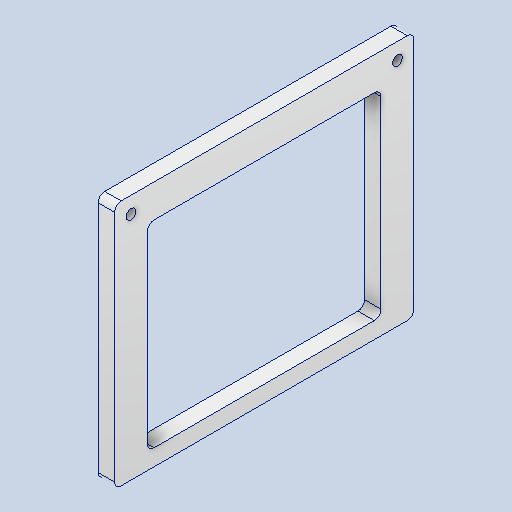
# Autodesk Inventor part: base_weel-v2-Plate-6
Saved by Autodesk Inventor 2025.2 (Build 292293000, 293)
## iProperties
Created: 2025-01-14
Part Number: base_weel-v2-Plate-6
Material: アルミニウム 6061
Document SubType Name: Modeling
Designer: haruy
Density: 2.7 g/cm^3
Appearance: アルミニウム - フラット
Author: haruy
Autodesk Inventor part; units mm, degrees
ref_plane "YZ Plane" through (0, 0, 0) normal (1, 0, 0) x (0, 1, 0)
ref_plane "XZ Plane" through (0, 0, 0) normal (0, 1, 0) x (-1, 0, 0)
ref_plane "XY Plane" through (0, 0, 0) normal (0, 0, 1) x (1, 0, 0)
sketch "スケッチ1" plane through (0, 0, 0) normal (1, 0, 0) x (0, 1, 0)
  line L0 (-222.6453, 335.6671) -> (407.3547, 335.6671)
  line L1 (407.3547, 335.6671) -> (407.3547, -294.3329)
  line L2 (407.3547, -294.3329) -> (-222.6453, -294.3329)
  line L3 (-222.6453, -294.3329) -> (-222.6453, 335.6671)
  line L4 (-222.6453, 335.6671) -> (407.3547, -294.3329) construction
  line L5 (407.3547, 335.6671) -> (-222.6453, -294.3329) construction
  line L6 (-202.6453, 238.6671) -> (-202.6453, -181.3329)
  line L7 (-202.6453, -181.3329) -> (-222.6453, -181.3329)
  line L8 (-222.6453, -181.3329) -> (-222.6453, 230.6671)
  line L9 (334.3547, 335.6671) -> (-149.6453, 335.6671)
  line L10 (-149.6453, 335.6671) -> (-149.6453, 315.6671)
  line L11 (-149.6453, 315.6671) -> (334.3547, 315.6671)
  line L12 (334.3547, 315.6671) -> (334.3547, 335.6671)
  line L13 (-202.6453, 238.6671) -> (-202.6453, 335.6671)
  line L14 (92.3547, 20.6671) -> (-864.2426, 20.6671)
  circle A0 centre (92.3547, 20.6671) radius 400
  line L15 (-237.6453, 45.6671) -> (-287.6453, 45.6671)
  line L16 (-287.6453, 45.6671) -> (-287.6453, -4.3329)
  line L17 (-287.6453, -4.3329) -> (-237.6453, -4.3329)
  line L18 (-237.6453, -4.3329) -> (-237.6453, 45.6671)
  line L19 (92.3547, 20.6671) -> (92.3547, -610.2507)
  line L20 (-222.6453, 60.6671) -> (-302.6453, 60.6671) construction
  line L21 (-302.6453, 60.6671) -> (-302.6453, 50.6671)
  line L22 (-302.6453, 50.6671) -> (-222.6453, 50.6671)
  line L23 (-222.6453, 50.6671) -> (-222.6453, 60.6671)
  line L24 (-302.6453, 50.6671) -> (-292.6453, 50.6671)
  line L25 (-292.6453, 50.6671) -> (-292.6453, 20.6671)
  line L26 (-292.6453, 20.6671) -> (-302.6453, 20.6671)
  line L27 (-302.6453, 20.6671) -> (-302.6453, 50.6671)
  line L28 (387.3547, 222.6671) -> (407.3547, 222.6671)
  line L29 (407.3547, 222.6671) -> (407.3547, -181.3329)
  line L30 (407.3547, -181.3329) -> (387.3547, -181.3329)
  line L31 (387.3547, -181.3329) -> (387.3547, 222.6671)
  line L32 (-129.8635, -294.3329) -> (334.3547, -294.3329)
  line L33 (334.3547, -294.3329) -> (334.3547, -274.3329)
  line L34 (334.3547, -274.3329) -> (-149.6453, -274.3329)
  line L35 (407.3547, 335.6671) -> (92.3547, 20.6671)
  line L36 (407.3547, 145.6671) -> (407.3547, 165.6671)
  circle A1 centre (604.3547, 20.6671) radius 122.5
  circle A2 centre (272.0452, 20.6671) radius 600
  circle A3 centre (634.0363, 20.6671) radius 200
  circle A4 centre (92.3547, 20.6671) radius 10
  arc A5 (92.3547, 170.6671) -> (92.3547, -129.3329) centre (92.3547, 20.6671) ccw
  arc A6 (92.3547, 160.6671) -> (92.3547, -119.3329) centre (92.3547, 20.6671) ccw
  line L37 (-53.9724, 53.6575) -> (-44.2173, 51.4581)
  line L38 (-45.2265, 58.3488) -> (-48.0856, 45.6671)
  line L39 (-48.0856, 45.6671) -> (-52.9632, 46.7668)
  line L40 (-52.9632, 46.7668) -> (-50.104, 59.4485)
  line L41 (-50.104, 59.4485) -> (-45.2265, 58.3488)
  arc A7 (63.2246, 162.7109) -> (63.2246, -121.3767) centre (92.3547, 20.6671) ccw
  circle A8 centre (-59.1356, 59.9471) radius 6.5
  circle A9 centre (-36.6854, 54.8855) radius 6.5 construction
  circle A10 centre (-36.6854, 54.8855) radius 1.5 construction
  circle A11 centre (-59.1356, 59.9471) radius 1.5
  line L42 (62.1879, 43.1671) -> (-81.7815, 43.1671)
  line L43 (-81.7815, 43.1671) -> (-81.7815, 28.1671)
  line L44 (-81.7815, 28.1671) -> (62.1879, 28.1671)
  line L45 (62.1879, 28.1671) -> (62.1879, 43.1671)
  line L46 (-53.9724, -12.3232) -> (-44.2173, -10.1239)
  line L47 (-45.2265, -17.0146) -> (-48.0856, -4.3329)
  line L48 (-48.0856, -4.3329) -> (-52.9632, -5.4326)
  line L49 (-52.9632, -5.4326) -> (-50.104, -18.1142)
  line L50 (-50.104, -18.1142) -> (-45.2265, -17.0146)
  circle A12 centre (-59.1356, -18.6128) radius 6.5
  circle A13 centre (-36.6854, -13.5513) radius 6.5 construction
  circle A14 centre (-36.6854, -13.5513) radius 1.5 construction
  circle A15 centre (-59.1356, -18.6128) radius 1.5
  line L51 (62.1879, -1.8329) -> (-81.7815, -1.8329)
  line L52 (-81.7815, -1.8329) -> (-81.7815, 13.1671)
  line L53 (-81.7815, 13.1671) -> (62.1879, 13.1671)
  line L54 (62.1879, 13.1671) -> (62.1879, -1.8329)
  line L55 (-59.1356, 59.9471) -> (-36.6854, 54.8855) construction
  line L56 (-36.6854, 54.8855) -> (-37.2352, 52.4467) construction
  line L57 (-37.2352, 52.4467) -> (-59.6855, 57.5083) construction
  line L58 (-59.6855, 57.5083) -> (-59.1356, 59.9471) construction
  line L59 (-36.6854, 54.8855) -> (-59.1356, 59.9471) construction
  line L60 (-59.1356, 59.9471) -> (-58.5858, 62.3858) construction
  line L61 (-58.5858, 62.3858) -> (-36.1355, 57.3243) construction
  line L62 (-36.1355, 57.3243) -> (-36.6854, 54.8855) construction
  line L63 (-36.1355, 57.3243) -> (-37.2352, 52.4467) construction
  line L64 (-37.2352, 52.4467) -> (-25.529, 49.8075) construction
  line L65 (-25.529, 49.8075) -> (-24.4294, 54.6851) construction
  line L66 (-24.4294, 54.6851) -> (-36.1355, 57.3243) construction
  line L67 (-58.5858, 62.3858) -> (-59.6855, 57.5083) construction
  line L68 (-59.6855, 57.5083) -> (-71.3917, 60.1475) construction
  line L69 (-71.3917, 60.1475) -> (-70.292, 65.0251) construction
  line L70 (-70.292, 65.0251) -> (-58.5858, 62.3858) construction
  line L71 (-62.9135, 65.9243) -> (-36.5865, 59.9887)
  line L72 (-36.5865, 59.9887) -> (-39.8855, 45.356)
  line L73 (-39.8855, 45.356) -> (-66.2126, 51.2916)
  line L74 (-66.2126, 51.2916) -> (-62.9135, 65.9243)
  line L75 (-62.9135, -24.5901) -> (-36.5865, -18.6545)
  line L76 (-36.5865, -18.6545) -> (-39.8855, -4.0218)
  line L77 (-39.8855, -4.0218) -> (-66.2126, -9.9574)
  line L78 (-66.2126, -9.9574) -> (-62.9135, -24.5901)
  arc A16 (-39.8855, 45.356) -> (-39.8855, -4.0218) centre (92.3547, 20.6671) ccw
  arc A17 (-66.2126, 51.2916) -> (-66.2126, -9.9574) centre (92.3547, 20.6671) ccw
  circle A18 centre (-60.1453, 35.6671) radius 1.25
  line L79 (-52.6453, 20.6671) -> (-52.6453, 95.4053)
  circle A19 centre (-45.1453, 35.6671) radius 1.25
  circle A20 centre (-60.1453, 5.6671) radius 1.25
  circle A21 centre (-45.1453, 5.6671) radius 1.25
  line L80 (92.3547, 20.6671) -> (92.3547, 160.6671)
  line L81 (92.3547, 20.6671) -> (44.4719, 152.2241)
  line L82 (92.3547, 160.6671) -> (92.3547, 170.6671)
  line L83 (-45.2298, 46.5609) -> (-41.9308, 61.1936)
  line L84 (-45.2298, -5.2267) -> (-41.9308, -19.8594)
  circle A22 centre (92.3547, 20.6671) radius 20
  line L85 (387.3547, 65.6671) -> (-202.6453, 65.6671)
  line L86 (-202.6453, 65.6671) -> (-202.6453, 45.6671)
  line L87 (-202.6453, 45.6671) -> (387.3547, 45.6671)
  line L88 (387.3547, 45.6671) -> (387.3547, 65.6671)
  line L89 (52.3547, 315.6671) -> (42.3547, 315.6671)
  line L90 (42.3547, 315.6671) -> (42.3547, 65.6671)
  line L91 (42.3547, 65.6671) -> (52.3547, 65.6671)
  line L92 (52.3547, 65.6671) -> (52.3547, 315.6671)
  line L93 (387.3547, -24.3329) -> (-202.6453, -24.3329)
  line L94 (-202.6453, -4.3329) -> (387.3547, -4.3329)
  line L95 (42.3547, -274.3329) -> (42.3547, -24.3329)
  line L96 (52.3547, -24.3329) -> (52.3547, -274.3329)
  line L97 (52.3547, 65.6671) -> (52.3547, -24.3329)
  line L98 (132.3547, 65.6671) -> (132.3547, -24.3329)
  circle A23 centre (112.3547, 55.6671) radius 1.5
  circle A24 centre (72.3547, 55.6671) radius 1.5
  circle A25 centre (112.3547, -14.3329) radius 1.5
  circle A26 centre (72.3547, -14.3329) radius 1.5
  circle A27 centre (47.3547, 145.6671) radius 1.5
  circle A28 centre (47.3547, 145.6671) radius 5
  circle A29 centre (-37.6453, 55.6671) radius 5
  circle A30 centre (-37.6453, 55.6671) radius 1.5
  line L99 (52.3547, 154.8312) -> (52.3547, 145.6671)
  line L100 (42.3547, 145.6671) -> (42.3547, 151.4341)
  line L101 (-45.395, 45.6671) -> (-35.2253, 51.2917)
  line L102 (-40.216, 65.6671) -> (-34.0112, 59.1013)
  circle A31 centre (47.3547, -104.3329) radius 1.5
  circle A32 centre (47.3547, -104.3329) radius 5
  circle A33 centre (-37.6453, -14.3329) radius 5
  circle A34 centre (-37.6453, -14.3329) radius 1.5
  line L103 (52.3547, -113.497) -> (52.3547, -104.3329)
  line L104 (42.3547, -104.3329) -> (42.3547, -110.0999)
  line L105 (-45.395, -4.3329) -> (-35.2253, -9.9575)
  line L106 (-40.216, -24.3329) -> (-34.0112, -17.7671)
  line L107 (-149.6453, -274.3329) -> (-149.6453, -294.3329)
  line L108 (334.3547, 335.6671) -> (314.3547, 335.6671)
  line L109 (314.3547, 335.6671) -> (314.3547, 315.6671)
  line L110 (314.3547, 315.6671) -> (334.3547, 315.6671)
  line L111 (334.3547, 315.6671) -> (334.3547, 335.6671)
  line L112 (334.3547, -294.3329) -> (314.3547, -294.3329)
  line L113 (314.3547, -294.3329) -> (314.3547, -274.3329)
  line L114 (314.3547, -274.3329) -> (334.3547, -274.3329)
  line L115 (334.3547, -274.3329) -> (334.3547, -294.3329)
  line L116 (289.3547, 315.6671) -> (387.3547, 217.6671)
  line L117 (387.3547, 217.6671) -> (376.7481, 207.0605)
  line L118 (376.7481, 207.0605) -> (278.7481, 305.0605)
  line L119 (278.7481, 305.0605) -> (289.3547, 315.6671)
  line L120 (289.3547, 315.6671) -> (289.3547, 335.6671)
  line L121 (290.2715, 314.7504) -> (279.6649, 304.1438)
  line L122 (290.625, 293.1836) -> (364.8712, 218.9374)
  line L123 (364.8712, 218.9374) -> (323.8591, 177.9252)
  line L124 (323.8591, 177.9252) -> (249.6128, 252.1714)
  line L125 (249.6128, 252.1714) -> (290.625, 293.1836)
  line L126 (383.256, 221.7658) -> (372.6494, 211.1592)
  line L127 (186.1172, 315.6671) -> (387.3547, 114.4295)
  line L128 (387.3547, 114.4295) -> (376.7481, 103.8229)
  line L129 (376.7481, 103.8229) -> (175.5105, 305.0605)
  line L130 (306.5349, 298.4869) -> (295.9283, 287.8803)
  line L131 (370.1745, 234.8473) -> (359.5679, 224.2407)
  circle A35 centre (292.0392, 302.376) radius 1.5
  circle A36 centre (306.1814, 288.2339) radius 1.5
  line L132 (278.7481, 305.0605) -> (268.1415, 315.6671)
  circle A37 centre (279.3547, 325.6671) radius 1.5
  circle A38 centre (269.3547, 325.6671) radius 1.5
  line L133 (264.3547, 335.6671) -> (264.3547, 315.6671)
  line L134 (186.1172, 315.6671) -> (186.1172, 315.6671)
  line L135 (186.1172, 315.6671) -> (186.1172, 335.6671)
  line L136 (175.5105, 305.0605) -> (164.9039, 315.6671)
  line L137 (161.1172, 335.6671) -> (161.1172, 315.6671)
  line L138 (376.7481, 207.0605) -> (387.3547, 196.4539)
  line L139 (387.3547, 217.6671) -> (407.3547, 217.6671)
  line L140 (387.3547, 114.4295) -> (387.3547, 114.4295)
  line L141 (376.7481, 103.8229) -> (387.3547, 93.2163)
  line L142 (-104.6453, 315.6671) -> (-202.6453, 217.6671)
  line L143 (-192.0387, 207.0605) -> (-94.0387, 305.0605)
  line L144 (-104.6453, 315.6671) -> (-104.6453, 335.6671)
  line L145 (-105.562, 314.7504) -> (-94.9554, 304.1438)
  line L146 (-180.1618, 218.9374) -> (-139.1496, 177.9252)
  line L147 (-64.9034, 252.1714) -> (-105.9156, 293.1836)
  line L148 (-198.5465, 221.7658) -> (-187.9399, 211.1592)
  line L149 (-1.4077, 315.6671) -> (-202.6453, 114.4295)
  line L150 (-202.6453, 114.4295) -> (-192.0387, 103.8229)
  line L151 (-192.0387, 103.8229) -> (9.1989, 305.0605)
  line L152 (9.1989, 305.0605) -> (-1.4077, 315.6671)
  line L153 (-121.8255, 298.4869) -> (-111.2189, 287.8803)
  line L154 (-94.0387, 305.0605) -> (-83.4321, 315.6671)
  line L155 (-79.6453, 335.6671) -> (-79.6453, 315.6671)
  line L156 (-1.4077, 315.6671) -> (-1.4077, 335.6671)
  line L157 (9.1989, 305.0605) -> (19.8055, 315.6671)
  line L158 (23.5923, 335.6671) -> (23.5923, 315.6671)
  line L159 (-192.0387, 207.0605) -> (-202.6453, 196.4539)
  line L160 (-202.6453, 217.6671) -> (-222.6453, 217.6671)
  line L161 (-192.0387, 103.8229) -> (-202.6453, 93.2163)
  line L162 (289.3547, -274.3329) -> (387.3547, -176.3329)
  line L163 (376.7481, -165.7263) -> (278.7481, -263.7263)
  line L164 (290.2715, -273.4161) -> (279.6649, -262.8095)
  line L165 (383.256, -180.4316) -> (372.6494, -169.825)
  line L166 (186.1172, -274.3329) -> (387.3547, -73.0953)
  line L167 (387.3547, -73.0953) -> (376.7481, -62.4887)
  line L168 (376.7481, -62.4887) -> (175.5105, -263.7263)
  line L169 (175.5105, -263.7263) -> (186.1172, -274.3329)
  line L170 (-1.4077, -274.3329) -> (-202.6453, -73.0953)
  line L171 (9.1989, -263.7263) -> (-1.4077, -274.3329)
  line L172 (-192.0387, -62.4887) -> (9.1989, -263.7263)
  line L173 (-202.6453, -73.0953) -> (-192.0387, -62.4887)
  line L174 (-192.0387, -165.7263) -> (-94.0387, -263.7263)
  line L175 (-104.6453, -274.3329) -> (-202.6453, -176.3329)
  line L176 (-105.562, -273.4161) -> (-94.9554, -262.8095)
  line L177 (-121.8255, -257.1527) -> (-111.2189, -246.5461)
  line L178 (-198.5465, -180.4316) -> (-187.9399, -169.825)
  line L179 (334.3547, 315.6671) -> (314.3547, 315.6671)
  arc A39 (92.3547, 106.6671) -> (92.3547, -65.3329) centre (92.3547, 20.6671) ccw construction
  circle A40 centre (1.4881, 69.1671) radius 21
  circle A41 centre (92.3547, 20.6671) radius 124
  circle A42 centre (1.4881, 69.1671) radius 17
  arc A43 (132.8499, 96.5364) -> (92.3547, 106.6671) centre (92.3547, 20.6671) ccw construction
  line L180 (52.3547, 65.6671) -> (42.3547, 65.6671)
  line L181 (42.3547, 65.6671) -> (42.3547, -24.3329)
  line L182 (42.3547, -24.3329) -> (52.3547, -24.3329)
  line L183 (52.3547, -24.3329) -> (52.3547, 65.6671)
  line L184 (52.3547, 315.6671) -> (42.3547, 315.6671)
  line L185 (42.3547, 315.6671) -> (42.3547, 335.6671)
  line L186 (42.3547, 335.6671) -> (52.3547, 335.6671)
  line L187 (52.3547, 335.6671) -> (52.3547, 315.6671)
  line L188 (52.3547, -274.3329) -> (42.3547, -274.3329)
  line L189 (42.3547, -274.3329) -> (42.3547, -294.3329)
  line L190 (42.3547, -294.3329) -> (52.3547, -294.3329)
  line L191 (52.3547, -294.3329) -> (52.3547, -274.3329)
  line L192 (142.3547, 315.6671) -> (142.3547, 65.6671)
  line L193 (132.3547, 65.6671) -> (132.3547, 315.6671)
  line L194 (142.3547, -274.3329) -> (142.3547, -24.3329)
  line L195 (132.3547, -24.3329) -> (132.3547, -274.3329)
  line L196 (142.3547, 65.6671) -> (142.3547, -24.3329)
  line L197 (132.3547, -24.3329) -> (132.3547, 65.6671)
  line L198 (142.3547, 315.6671) -> (142.3547, 335.6671)
  line L199 (132.3547, 335.6671) -> (132.3547, 315.6671)
  line L200 (142.3547, -274.3329) -> (142.3547, -294.3329)
  line L201 (132.3547, -294.3329) -> (132.3547, -274.3329)
  line L202 (51.9456, 143.6861) -> (57.3547, 156.2215)
  line L203 (43.613, 142.3505) -> (37.3547, 149.411)
  line L204 (51.9456, -102.3519) -> (57.3547, -114.8873)
  line L205 (43.613, -101.0163) -> (37.3547, -108.0768)
  arc A44 (132.8499, 96.5364) -> (51.8596, -55.2021) centre (92.3547, 20.6671) ccw
  circle A45 centre (92.3547, 20.6671) radius 86 construction
  circle A46 centre (92.3547, 20.6671) radius 78.5
  circle A47 centre (47.3547, 78.6671) radius 1.5
  circle A48 centre (47.3547, 78.6671) radius 5
  circle A49 centre (137.3547, 78.6671) radius 5
  circle A50 centre (137.3547, 78.6671) radius 1.5
  line L206 (138.9096, 73.915) -> (147.3547, 76.6783)
  line L207 (132.6797, 76.8939) -> (127.3547, 90.9327)
  line L208 (142.3547, 81.1836) -> (142.3547, 90.6385)
  arc A51 (142.3547, 90.6385) -> (132.8499, 96.5364) centre (92.3547, 20.6671) ccw
  line L209 (52.0297, 76.8939) -> (57.3547, 90.9327)
  line L210 (45.7999, 73.915) -> (37.3547, 76.6783)
  circle A52 centre (47.3547, -37.3329) radius 1.5
  circle A53 centre (47.3547, -37.3329) radius 5
  line L211 (52.0297, -35.5596) -> (57.3547, -49.5985) construction
  line L212 (45.7999, -32.5808) -> (37.3547, -35.344)
  line L213 (52.3547, -46.8773) -> (52.3547, -55.4643)
  arc A54 (51.8288, -55.1857) -> (52.3547, -55.4643) centre (92.3547, 20.6671) ccw
  line L214 (52.3547, -55.4643) -> (52.3547, -37.3329)
  line L215 (315.0202, 290.0016) -> (304.4136, 279.395)
  line L216 (387.3547, 217.6671) -> (407.3547, 217.6671)
  line L217 (386.438, 218.5839) -> (375.8314, 207.9773)
  circle A55 centre (374.0636, 220.3516) radius 1.5
  circle A56 centre (359.9215, 234.4938) radius 1.5
  circle A57 centre (397.3547, 207.6671) radius 1.5
  circle A58 centre (397.3547, 197.6671) radius 1.5
  line L218 (407.3547, 192.6671) -> (387.3547, 192.6671)
  line L219 (361.6893, 243.3326) -> (351.0827, 232.726)
  circle A59 centre (176.1172, 325.6671) radius 1.5
  circle A60 centre (166.1172, 325.6671) radius 1.5
  line L220 (290.2715, 314.7504) -> (187.0339, 314.7504)
  line L221 (279.6649, 304.1438) -> (176.4273, 304.1438)
  line L222 (187.0339, 314.7504) -> (176.4273, 304.1438)
  circle A61 centre (188.8017, 302.376) radius 1.5
  circle A62 centre (202.9438, 288.2339) radius 1.5
  line L223 (211.7826, 290.0016) -> (201.176, 279.395)
  line L224 (387.3547, 114.4295) -> (407.3547, 114.4295)
  line L225 (407.3547, 89.4295) -> (387.3547, 89.4295)
  circle A63 centre (397.3547, 104.4295) radius 1.5
  circle A64 centre (397.3547, 94.4295) radius 1.5
  line L226 (386.438, 115.3463) -> (375.8314, 104.7397)
  circle A65 centre (374.0636, 117.114) radius 1.5
  circle A66 centre (359.9215, 131.2562) radius 1.5
  line L227 (361.6893, 140.095) -> (351.0827, 129.4884)
  line L228 (-104.6453, 315.6671) -> (-104.6453, 335.6671)
  line L229 (-105.562, 314.7504) -> (-94.9554, 304.1438)
  line L230 (-121.8255, 298.4869) -> (-111.2189, 287.8803)
  circle A67 centre (-107.3298, 302.376) radius 1.5
  circle A68 centre (-121.4719, 288.2339) radius 1.5
  circle A69 centre (-94.6453, 325.6671) radius 1.5
  circle A70 centre (-84.6453, 325.6671) radius 1.5
  line L231 (-79.6453, 335.6671) -> (-79.6453, 315.6671)
  line L232 (-1.4077, 315.6671) -> (-1.4077, 335.6671)
  line L233 (23.5923, 335.6671) -> (23.5923, 315.6671)
  line L234 (-202.6453, 217.6671) -> (-222.6453, 217.6671)
  line L235 (-130.3107, 290.0016) -> (-119.7041, 279.395)
  line L236 (-176.9798, 243.3326) -> (-166.3732, 232.726)
  circle A71 centre (-175.212, 234.4938) radius 1.5
  circle A72 centre (-189.3542, 220.3516) radius 1.5
  line L237 (-201.7285, 218.5839) -> (-191.1219, 207.9773)
  line L238 (-222.6453, 192.6671) -> (-202.6453, 192.6671)
  circle A73 centre (-212.6453, 197.6671) radius 1.5
  circle A74 centre (-212.6453, 207.6671) radius 1.5
  circle A75 centre (8.5923, 325.6671) radius 1.5
  circle A76 centre (18.5923, 325.6671) radius 1.5
  line L239 (-2.3244, 314.7504) -> (8.2822, 304.1438)
  circle A77 centre (-4.0922, 302.376) radius 1.5
  circle A78 centre (-18.2343, 288.2339) radius 1.5
  line L240 (-27.0731, 290.0016) -> (-16.4665, 279.395)
  line L241 (-202.6453, 114.4295) -> (-222.6453, 114.4295)
  line L242 (-222.6453, 89.4295) -> (-202.6453, 89.4295)
  circle A79 centre (-212.6453, 94.4295) radius 1.5
  circle A80 centre (-212.6453, 104.4295) radius 1.5
  line L243 (-201.7285, 115.3463) -> (-191.1219, 104.7397)
  circle A81 centre (-189.3542, 117.114) radius 1.5
  circle A82 centre (-175.212, 131.2562) radius 1.5
  line L244 (-176.9798, 140.095) -> (-166.3732, 129.4884)
  line L245 (289.3547, -274.3329) -> (289.3547, -294.3329)
  line L246 (290.2715, -273.4161) -> (279.6649, -262.8095)
  circle A83 centre (292.0392, -261.0418) radius 1.5
  circle A84 centre (306.1814, -246.8996) radius 1.5
  circle A85 centre (279.3547, -284.3329) radius 1.5
  circle A86 centre (269.3547, -284.3329) radius 1.5
  line L247 (264.3547, -294.3329) -> (264.3547, -274.3329)
  line L248 (186.1172, -274.3329) -> (186.1172, -294.3329)
  line L249 (161.1172, -294.3329) -> (161.1172, -274.3329)
  line L250 (387.3547, -176.3329) -> (407.3547, -176.3329)
  line L251 (-104.6453, -274.3329) -> (-104.6453, -294.3329)
  line L252 (-79.6453, -294.3329) -> (-79.6453, -274.3329)
  line L253 (23.5923, -294.3329) -> (23.5923, -274.3329)
  line L254 (-105.562, -273.4161) -> (-94.9554, -262.8095)
  line L255 (-202.6453, -176.3329) -> (-222.6453, -176.3329)
  line L256 (315.0202, -248.6674) -> (304.4136, -238.0608)
  line L257 (361.6893, -201.9984) -> (351.0827, -191.3918)
  circle A87 centre (359.9215, -193.1595) radius 1.5
  circle A88 centre (374.0636, -179.0174) radius 1.5
  line L258 (386.438, -177.2496) -> (375.8314, -166.643)
  line L259 (407.3547, -151.3329) -> (387.3547, -151.3329)
  circle A89 centre (397.3547, -156.3329) radius 1.5
  circle A90 centre (397.3547, -166.3329) radius 1.5
  circle A91 centre (176.1172, -284.3329) radius 1.5
  circle A92 centre (166.1172, -284.3329) radius 1.5
  line L260 (187.0339, -273.4161) -> (176.4273, -262.8095)
  circle A93 centre (188.8017, -261.0418) radius 1.5
  circle A94 centre (202.9438, -246.8996) radius 1.5
  line L261 (211.7826, -248.6674) -> (201.176, -238.0608)
  line L262 (387.3547, -73.0953) -> (407.3547, -73.0953)
  line L263 (407.3547, -48.0953) -> (387.3547, -48.0953)
  circle A95 centre (397.3547, -53.0953) radius 1.5
  circle A96 centre (397.3547, -63.0953) radius 1.5
  line L264 (386.438, -74.012) -> (375.8314, -63.4054)
  circle A97 centre (374.0636, -75.7798) radius 1.5
  circle A98 centre (359.9215, -89.9219) radius 1.5
  line L265 (361.6893, -98.7608) -> (351.0827, -88.1542)
  circle A99 centre (-84.6453, -284.3329) radius 1.5
  circle A100 centre (-94.6453, -284.3329) radius 1.5
  circle A101 centre (-107.3298, -261.0418) radius 1.5
  circle A102 centre (-121.4719, -246.8996) radius 1.5
  line L266 (-130.3107, -248.6674) -> (-119.7041, -238.0608)
  circle A103 centre (-175.212, -193.1595) radius 1.5
  line L267 (-176.9798, -201.9984) -> (-166.3732, -191.3918)
  circle A104 centre (-189.3542, -179.0174) radius 1.5
  line L268 (-201.7285, -177.2496) -> (-191.1219, -166.643)
  circle A105 centre (-212.6453, -166.3329) radius 1.5
  circle A106 centre (-212.6453, -156.3329) radius 1.5
  line L269 (-222.6453, -151.3329) -> (-202.6453, -151.3329)
  line L270 (-202.6453, -73.0953) -> (-222.6453, -73.0953)
  line L271 (-222.6453, -48.0953) -> (-202.6453, -48.0953)
  circle A107 centre (-212.6453, -53.0953) radius 1.5
  circle A108 centre (-212.6453, -63.0953) radius 1.5
  line L272 (-201.7285, -74.012) -> (-191.1219, -63.4054)
  circle A109 centre (-189.3542, -75.7798) radius 1.5
  circle A110 centre (-175.212, -89.9219) radius 1.5
  line L273 (-176.9798, -98.7608) -> (-166.3732, -88.1542)
  line L274 (-27.0731, -248.6674) -> (-16.4665, -238.0608)
  circle A111 centre (-18.2343, -246.8996) radius 1.5
  circle A112 centre (-4.0922, -261.0418) radius 1.5
  line L275 (-2.3244, -273.4161) -> (8.2822, -262.8095)
  line L276 (-1.4077, -274.3329) -> (-1.4077, -294.3329)
  circle A113 centre (18.5923, -284.3329) radius 1.5
  circle A114 centre (8.5923, -284.3329) radius 1.5
  line L277 (-202.6453, 222.6671) -> (-222.6453, 222.6671)
  line L278 (357.3547, 65.6671) -> (357.3547, 45.6671)
  circle A115 centre (367.3547, 55.6671) radius 1.5
  circle A116 centre (377.3547, 55.6671) radius 1.5
  circle A117 centre (397.3547, 55.6671) radius 1.5
  circle A118 centre (397.3547, 45.6671) radius 1.5
  line L279 (387.3547, 45.6671) -> (407.3547, 45.6671)
  line L280 (357.3547, -24.3329) -> (357.3547, -4.3329)
  circle A119 centre (367.3547, -14.3329) radius 1.5
  circle A120 centre (377.3547, -14.3329) radius 1.5
  circle A121 centre (397.3547, -14.3329) radius 1.5
  circle A122 centre (397.3547, -4.3329) radius 1.5
  line L281 (-172.6453, 65.6671) -> (-172.6453, 45.6671)
  circle A123 centre (-182.6453, 55.6671) radius 1.5
  circle A124 centre (-192.6453, 55.6671) radius 1.5
  circle A125 centre (-212.6453, 55.6671) radius 1.5
  circle A126 centre (-212.6453, 45.6671) radius 1.5
  line L282 (-172.6453, -24.3329) -> (-172.6453, -4.3329)
  circle A127 centre (-182.6453, -14.3329) radius 1.5
  circle A128 centre (-192.6453, -14.3329) radius 1.5
  circle A129 centre (-212.6453, -14.3329) radius 1.5
  circle A130 centre (-212.6453, -4.3329) radius 1.5
  circle A131 centre (140.3547, 365.6671) radius 44
  circle A132 centre (42.3547, 365.6671) radius 44
  circle A133 centre (42.3547, 365.6671) radius 15
  line L283 (387.3547, 65.6671) -> (407.3547, 65.6671)
  line L284 (387.3547, 35.6671) -> (407.3547, 35.6671)
  line L285 (-222.6453, 66.1671) -> (-297.6453, 66.1671)
  line L286 (-297.6453, 66.1671) -> (-297.6453, 20.6671)
  line L287 (-297.6453, 20.6671) -> (-222.6453, 20.6671)
  line L288 (-222.6453, 20.6671) -> (-222.6453, 66.1671)
  circle A134 centre (-212.6453, 68.6671) radius 1.5
  line L289 (-222.6453, -24.8329) -> (-297.6453, -24.8329)
  line L290 (-297.6453, -24.8329) -> (-297.6453, 20.6671)
  circle A135 centre (-282.6453, 40.6671) radius 1.5
  circle A136 centre (-242.6453, 0.6671) radius 1.5
  line L291 (-237.6453, 45.6671) -> (-287.6453, -4.3329)
  line L292 (-287.6453, 45.6671) -> (-237.6453, -4.3329)
  line L293 (-292.6453, 50.6671) -> (-292.6453, 66.1671)
  line L294 (-222.6453, 56.1671) -> (-292.6453, 56.1671)
  line L295 (-292.6453, -9.3329) -> (-292.6453, -24.8329)
  line L296 (-292.6453, -9.3329) -> (-292.6453, 20.6671)
  line L297 (-222.6453, -14.8329) -> (-292.6453, -14.8329)
  line L298 (-287.6453, 45.6671) -> (-292.6453, 50.6671)
  line L299 (-237.6453, 45.6671) -> (-232.6453, 50.6671)
  line L300 (-237.6453, -4.3329) -> (-232.6453, -9.3329)
  line L301 (-287.6453, -4.3329) -> (-292.6453, -9.3329)
  line L302 (-235.678, -13.3713) -> (-241.1808, -7.8684)
  line L303 (-241.1808, -7.8684) -> (-291.1808, 42.1316)
  line L304 (-291.1808, 42.1316) -> (-297.6453, 48.596)
  line L305 (-297.6453, 48.596) -> (-297.6453, 66.1671)
  line L306 (-296.1808, -5.7973) -> (-291.1808, -0.7973)
  line L307 (-291.1808, -0.7973) -> (-241.1808, 49.2027)
  line L308 (-241.1808, 49.2027) -> (-236.1809, 54.2025)
  line L309 (-297.6453, -19.8329) -> (-208.1792, -19.8329) construction
  line L310 (-229.6126, -5.2945) -> (-234.1097, -0.7973)
  line L311 (-234.1097, -0.7973) -> (-284.1097, 49.2027)
  line L312 (-284.1097, 49.2027) -> (-287.6453, 52.7382)
  line L313 (-287.6453, 52.7382) -> (-287.6453, 66.1671)
  line L314 (-289.1097, -12.8684) -> (-284.1097, -7.8684)
  line L315 (-284.1097, -7.8684) -> (-234.1097, 42.1316)
  line L316 (-234.1097, 42.1316) -> (-229.1097, 47.1316)
  line L317 (-232.6453, 66.1671) -> (-232.6453, -19.8329)
  line L318 (-229.1097, 47.1316) -> (-232.6453, 43.596)
  line L319 (-236.1809, 54.2025) -> (-234.2163, 56.1671)
  line L320 (-287.6453, 52.7382) -> (-291.0742, 56.1671)
  line L321 (-289.1097, -12.8684) -> (-291.0742, -14.8329)
  line L322 (-229.6126, -5.2945) -> (-232.6453, -2.2618)
  line L323 (-235.678, -13.3713) -> (-234.2163, -14.8329)
  circle A137 centre (-227.6453, 61.1671) radius 5
  circle A138 centre (-227.6453, 61.1671) radius 1.5
  circle A139 centre (-227.6453, -19.8329) radius 1.5
  point P0 (0, 0)
  point P1 (-49.0948, 52.5578)
  point P2 (-36.6854, 54.8855)
  point P3 (-57.6453, 20.6671)
  point P4 (-149.6453, 325.6671)
  point P5 (-202.6453, 114.4295)
  point P6 (-69.1428, 20.6671)
  point P7 (397.3547, 45.6671)
  point P8 (387.3547, 55.6671)
  point P9 (-292.6453, 43.596)
  point P10 (-269.7163, 20.6671)
  point P11 (-292.6453, -2.2618)
  point P12 (-262.6453, 27.7382)
  point P13 (-255.5742, 20.6671)
  point P14 (-232.6453, 43.596)
  point P15 (-262.6453, 13.596)
  point P16 (-232.6453, 56.1671)
  point P17 (-232.6453, -14.8329)
  dimension "d0" = 3
  dimension "d1" = 5
  dimension "d2" = 5
  dimension "d3" = 3
  dimension "d4" = 5
  dimension "d5" = 5
  dimension "d6" = 10
  dimension "d7" = 5
  dimension "d8" = 5
  dimension "d9" = 5
  dimension "d10" = 5
  dimension "d11" = 10
  dimension "d12" = 10
  dimension "d13" = 3
  constraints: 644 end point, 139 centre point, 18 point on circle, 15 point on line, 8 symmetric about line, 4 collinear, 3 coincident, 2 perpendicular, 2 tangent, 2 vertical, 1 parallel, 25 other
  measures "d0" diameter of A135
  measures "d1" distance from line of A135.centre L16
  measures "d2" distance from line of A135.centre L15
  measures "d3" diameter of A136
  measures "d4" distance from line of A136.centre L18
  measures "d5" distance from line of L17 A136.centre
  measures "d6" distance between parallel lines of L285 L294
  measures "d7" distance between parallel lines of L292 L303
  measures "d8" distance between parallel lines of L291 L307
  measures "d9" distance between parallel lines of L292 L311
  measures "d10" distance between parallel lines of L291 L315
  measures "d11" distance between parallel lines of L317 L8
  measures "d12" diameter of A137
  measures "d13" diameter of A138
extrude "押し出し1" add sketch "スケッチ1" against normal blind 5 contours L286 L304 L25 L14 | L14 L296 L295 L289 L290 | L286 L22 L25 L304 | L286 L285 L293 L22 | L295 L297 L3 L289 | L293 L285 L313 L294 | L3 A137 L285 | L297 L317 L14 L3 | L285 L317 L294 L313 | A137 | L3 L294 A137 | A137 L317 L285 | L14 L317 L22 L3 | L317 L294 L3 L22 | L294 L317 A137
fillet "フィレット1" radius 2 8 edges at (-2.5, -297.6453, 66.1671) (-2.5, -222.6453, 66.1671) (-2.5, -222.6453, -24.8329) (-2.5, -297.6453, -24.8329) (-2.5, -292.6453, -14.8329) (-2.5, -232.6453, -14.8329) (-2.5, -232.6453, 56.1671) (-2.5, -292.6453, 56.1671)
equation "\"d2\" = d1"
equation "\"d5\" = d4"
